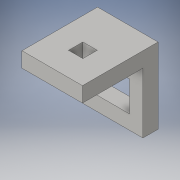
# Autodesk Inventor part: l braket w. squares
Saved by Autodesk Inventor 2016 (Build 200138000, 138)
## iProperties
Created: 2016-01-16
Part Number: l braket w. squares
Material: Generic
Document SubType Name: Modeling
Designer: Administrator
Density: 1 g/cm^3
Appearance: Default
Author: Administrator
Autodesk Inventor part; units mm, degrees
ref_plane "YZ Plane" through (0, 0, 0) normal (1, 0, 0) x (0, 1, 0)
ref_plane "XZ Plane" through (0, 0, 0) normal (0, 1, 0) x (-1, 0, 0)
ref_plane "XY Plane" through (0, 0, 0) normal (0, 0, 1) x (1, 0, 0)
sketch "Sketch1" plane through (0, 0, 0) normal (0, 1, 0) x (-1, 0, 0)
  line L0 (0, 0) -> (25.4, 0)
  line L1 (25.4, 0) -> (25.4, 25.4)
  line L2 (25.4, 25.4) -> (0, 25.4)
  line L3 (0, 25.4) -> (0, 0)
  dimension "d0" = 25.4
  dimension "d1" = 25.4
  constraints: 8 end point, 2 parallel, 1 horizontal, 1 perpendicular
  measures "d0" distance of L2.end L1.end
  measures "d1" distance of L1.end L0.end
extrude "Extrusion1" add sketch "Sketch1" along normal blind 6.35
sketch "Sketch2" plane through (0, 6.35, 0) normal (0, 1, 0) x (1, 0, 0)
  line L0 (0, 0) -> (-25.4, 0) projected
  line L1 (0, 0) -> (-25.4, 0)
  line L2 (-25.4, 0) -> (-25.4, 6.35)
  line L3 (-25.4, 6.35) -> (0, 6.35)
  line L4 (0, 6.35) -> (0, 0)
  dimension "d4" = 6.35
  constraints: 8 end point, 2 parallel, 1 horizontal, 1 perpendicular
  measures "d4" distance of L1.end L2.end
extrude "Extrusion2" add sketch "Sketch2" against normal blind 31.75
sketch "Sketch3" plane through (-25.4, 0, 0) normal (0, 0, 1) x (1, 0, 0)
  line L0 (5.1775, -6.7435) -> (19.8333, -6.7435)
  line L1 (19.8333, -6.7435) -> (19.8333, -19.4435)
  line L2 (19.8333, -19.4435) -> (5.1775, -19.4435)
  line L3 (5.1775, -19.4435) -> (5.1775, -6.7435)
  line L4 (5.1775, -6.7435) -> (19.8333, -19.4435) construction
  line L5 (19.8333, -6.7435) -> (5.1775, -19.4435) construction
  point P0 (25.4, 0)
  point P1 (12.5054, -13.0935)
  dimension "d7" = 14.6558
  dimension "d8" = 12.7
  constraints: 12 end point, 2 midpoint, 2 parallel, 1 horizontal, 1 perpendicular
  measures "d7" distance of L1.end L2.end
  measures "d8" distance of L0.end L1.end
extrude "Extrusion3" cut sketch "Sketch3" against normal blind 31.75
sketch "Sketch4" plane through (0, 0, 0) normal (0, -1, 0) x (1, 0, 0)
  line L0 (-15.7889, 15.4698) -> (-9.7437, 15.4698)
  line L1 (-9.7437, 15.4698) -> (-9.7437, 9.4246)
  line L2 (-9.7437, 9.4246) -> (-15.7889, 9.4246)
  line L3 (-15.7889, 9.4246) -> (-15.7889, 15.4698)
  line L4 (-15.7889, 15.4698) -> (-9.7437, 9.4246) construction
  line L5 (-9.7437, 15.4698) -> (-15.7889, 9.4246) construction
  point P0 (0, 0)
  point P1 (-12.7663, 12.4472)
  dimension "d11" = 6.0452
  dimension "d12" = 6.0452
  constraints: 12 end point, 2 midpoint, 2 parallel, 1 horizontal, 1 perpendicular
  measures "d11" distance of L1.end L2.end
  measures "d12" distance of L0.end L1.end
extrude "Extrusion4" cut sketch "Sketch4" against normal blind 25.4
body "Solid1"
